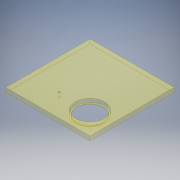
# Autodesk Inventor part: cote droit
Saved by Autodesk Inventor 2018.1 (Build 221171000, 171)
## iProperties
Created: 2022-06-30
Part Number: cote droit
Material: Generic
Document SubType Name: Modeling
Designer: Bureau
Density: 1 g/cm^3
Appearance: Default
Author: Bureau
Autodesk Inventor part; units mm, degrees
ref_plane "YZ Plane" through (0, 0, 0) normal (1, 0, 0) x (0, 1, 0)
ref_plane "XZ Plane" through (0, 0, 0) normal (0, 1, 0) x (-1, 0, 0)
ref_plane "XY Plane" through (0, 0, 0) normal (0, 0, 1) x (1, 0, 0)
sketch "Sketch1" plane through (0, 0, 0) normal (0, 0, 1) x (1, 0, 0)
  line L0 (0, 0) -> (150, 0)
  line L1 (150, 0) -> (150, 150)
  line L2 (150, 150) -> (0, 150)
  line L3 (0, 150) -> (0, 0)
  dimension "d0" = 150
  dimension "d1" = 150
  constraints: 8 end point, 3 perpendicular, 1 horizontal
  measures "d0" distance of L0.start L0.end
  measures "d1" distance of L0.end L1.end
extrude "Extrusion1" add sketch "Sketch1" along normal blind 8
sketch "Sketch2" plane through (0, 0, 8) normal (0, 0, 1) x (1, 0, 0)
  circle A0 centre (110, 40) radius 24
  line L0 (0, 0) -> (150, 0) projected
  line L1 (150, 0) -> (150, 150) projected
  line L2 (110, 40) -> (55, 40)
  circle A1 centre (55, 40) radius 2
  dimension "d4" = 48
  dimension "d5" = 40
  dimension "d6" = 40
  dimension "d7" = 55
  dimension "d8" = 4
  constraints: 2 centre point, 2 end point, 1 coincident, 1 horizontal
  measures "d4" diameter of A0
  measures "d5" distance from line of L0 L2.start
  measures "d6" distance from line of L1 L2.start
  measures "d7" distance of L2.start L2.end
  measures "d8" diameter of A1
extrude "Extrusion2" cut sketch "Sketch2" against normal blind 8
sketch "Sketch3" plane through (0, 0, 8) normal (0, 0, 1) x (1, 0, 0)
  circle A0 centre (110, 40) radius 26
  point P0 (0, 0)
  dimension "d12" = 52
  constraints: 1 centre point
  measures "d12" diameter of A0
extrude "Extrusion3" cut sketch "Sketch3" against normal blind 7
body "Solid1"
